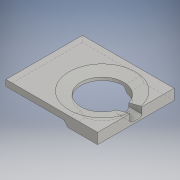
# Autodesk Inventor part: wide_access_platform_v01_ok
Saved by Autodesk Inventor 2016 (Build 200138000, 138)
## iProperties
Created: 2016-07-30
Part Number: wide_access_platform_v01_ok
Material: Generic
Document SubType Name: Modeling
Designer: stephenholtz
Density: 1 g/cm^3
Appearance: Default
Author: stephenholtz
Autodesk Inventor part; units mm, degrees
ref_plane "YZ Plane" through (0, 0, 0) normal (1, 0, 0) x (0, 1, 0)
ref_plane "XZ Plane" through (0, 0, 0) normal (0, 1, 0) x (-1, 0, 0)
ref_plane "XY Plane" through (0, 0, 0) normal (0, 0, 1) x (1, 0, 0)
sketch "Sketch1" plane through (0, 0, 0) normal (0, 1, 0) x (-1, 0, 0)
  line L0 (12.5, 15) -> (-12.5, 15)
  line L1 (-12.5, 15) -> (-12.5, -15)
  line L2 (-12.5, -15) -> (12.5, -15)
  line L3 (12.5, -15) -> (12.5, 15)
  line L4 (12.5, 15) -> (-12.5, -15) construction
  line L5 (-12.5, 15) -> (12.5, -15) construction
  point P0 (0, 0)
  dimension "d0" = 25
  dimension "d1" = 30
  constraints: 12 end point, 2 midpoint, 2 parallel, 1 horizontal, 1 perpendicular
  measures "d0" distance of L2.end L1.end
  measures "d1" distance of L1.end L0.end
extrude "Extrusion1" add sketch "Sketch1" along normal blind 4
sketch "Sketch2" plane through (0, 4, 0) normal (0, 1, 0) x (1, 0, 0)
  line L0 (-12.5, 15) -> (-12.5, -15) construction
  line L1 (-12.5, -11) -> (12.5, -11) construction
  line L2 (12.5, -15) -> (12.5, 15) construction
  line L3 (-12.5, -15) -> (12.5, -15) construction
  circle A0 centre (0, -4) radius 7
  line L4 (0, -15) -> (0, 15) construction
  line L5 (12.5, 15) -> (-12.5, 15) construction
  point P0 (0, 0)
  point P1 (0, -11)
  dimension "d5" = 14
  dimension "d4" = 4
  constraints: 4 end point, 3 midpoint, 3 point on line, 1 horizontal, 1 vertical alignment, 2 other
  measures "d4" distance between parallel lines of L3 L1
extrude "Extrusion2" cut sketch "Sketch2" against normal through all
sketch "Sketch3" plane through (0, 0, 0) normal (1, 0, 0) x (0, 1, 0)
  line L0 (4, -3) -> (4, 11) construction
  line L1 (0, -15) -> (0, 15) construction
  line L2 (0, 15) -> (4, 15) construction
  line L3 (4, -15) -> (4, 15) construction
  line L4 (0, -15) -> (4, -15) construction
  line L5 (4, 4) -> (0, 4) construction
  line L6 (2, 4) -> (0.5, 5.258649)
  line L7 (2, 4) -> (2, -15)
  line L8 (0, -15) -> (4, -15)
  line L9 (2, -15) -> (1.618278, -15)
  line L10 (0.5, 15) -> (0.5, 5.258649)
  line L11 (1.618278, -15) -> (0, -15)
  line L12 (0, -15) -> (0, 15)
  line L13 (0, 15) -> (0.5, 15)
  line L14 (0, 15) -> (4, 15)
  line L15 (4, 11) -> (0, 11)
  line L16 (4, -3) -> (0, -3)
  point P0 (0, 0)
  dimension "d6" = 50
  dimension "d7" = 2
  dimension "d8" = 1.5
  constraints: 16 end point, 3 collinear, 3 perpendicular, 3 point on line, 2 midpoint, 1 parallel
  measures "d6" angle of L7 L6
  measures "d7" distance between parallel lines of L1 L7
  measures "d8" distance between parallel lines of L7 L10
extrude "Extrusion3" cut sketch "Sketch3" along normal through all both and the other way through all
sketch "Sketch7" plane through (-12.5, 4, 15) normal (0, 0, 1) x (1, 0, 0)
  line L0 (0, -3.5) -> (25, -3.5) construction
  line L1 (25, -3.5) -> (25, 0) construction
  line L2 (0, 0) -> (25, 0) construction
  line L3 (0, -3.5) -> (0, 0) construction
  line L4 (5.5, -2) -> (19.5, -2) construction
  circle A0 centre (12.5, -2) radius 0.875 construction
  line L5 (12.5, -2) -> (14.5, -2) construction
  line L6 (12.5, 0) -> (12.5, -3.5) construction
  line L7 (12.5, -2) -> (10.5, -2) construction
  spline S0 degree 5 poles (10.5, -2) (10.5, -1.67732) (11.1, -1.13952) (13.34, -0.733036) (15.98, -2) (13.34, -3.266964) (11.1, -2.86048) (10.5, -2.32268) (10.5, -2) knots 0 0 0 0 0 0 0.3 0.5 0.7 1 1 1 1 1 1
  line L8 (10.5, -2) -> (10.5, 0)
  line L9 (14.5, -2) -> (14.5, 0)
  line L10 (10.5, 0) -> (14.5, 0)
  point P0 (12.5, -4)
  point P1 (12.5, -2.875)
  dimension "d26" = 1.75
  dimension "d27" = 2
  dimension "d28" = 2
  constraints: 12 end point, 6 point on line, 3 coincident, 3 midpoint, 2 perpendicular, 2 point on circle, 1 centre point, 1 collinear, 4 other
  measures "d26" diameter of A0
  measures "d27" distance of L5.end L5.start
  measures "d28" distance of point (12.5, -2) L7.end
extrude "Extrusion4" cut sketch "Sketch7" against normal blind 10.25
sketch "Sketch4" plane through (0, 0, 0) normal (1, 0, 0) x (0, 1, 0)
  line L0 (2, -15) -> (2, 4)
  line L1 (2, 4) -> (0.5, 5.258649)
  line L2 (0.5, 5.258649) -> (0.5, 15)
  line L3 (0.5, 15) -> (4, 15)
  line L4 (4, -15) -> (4, 15)
  line L5 (2, -15) -> (4, -15)
  line L6 (4, 11) -> (4, -3)
  line L7 (2, 4) -> (2, -15)
  line L8 (4, 4) -> (0, 4)
  line L9 (4, -15) -> (4, 15)
  line L10 (2, 4.5) -> (2, 3.5)
  line L11 (2.965926, 4.758819) -> (1.034074, 4.241181)
  line L12 (1.034074, 4.241181) -> (6.725631, -17)
  line L13 (6.725631, -17) -> (8.657483, -16.482362)
  line L14 (8.657483, -16.482362) -> (3.169251, 4)
  line L15 (3.169251, 4) -> (1.098698, 4)
  point P0 (0, 0)
  point P1 (2, 4)
  dimension "d13" = 0.5
  dimension "d18" = 15
  dimension "d19" = 2
  dimension "d20" = 2
  constraints: 15 end point, 4 midpoint, 3 point on line, 2 parallel, 2 perpendicular, 1 collinear
  measures "d13" distance of L10.start L0.end
  measures "d18" angle of L8 L11
  measures "d19" distance between parallel lines of L12 L14
  measures "d20" vertical distance of L4.start L12.end
revolve "Revolution2" cut sketch "Sketch4" angle 360 about axis through (0, 4, 4) along (0, -1, 0) contours L0 L12 L8 | L0 L8 L14 L4 L12 | L4 L14 L13 L12
body "Solid1"
